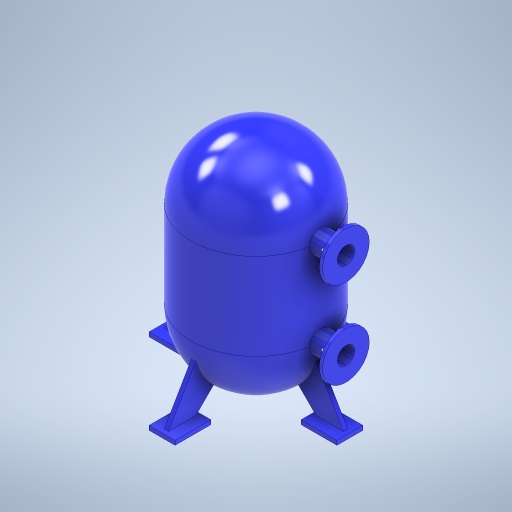
# Autodesk Inventor part: Tank
Saved by Autodesk Inventor 2023 (Build 270158000, 158)
## iProperties
Created: 2024-11-19
Part Number: Tank
Material: Generisch
Document SubType Name: Modeling
Designer: aurich
Density: 1 g/cm^3
Appearance: Vorgabe
Author: aurich
Autodesk Inventor part; units mm, degrees
ref_plane "XZ Plane" through (0, 0, 0) normal (0, 1, 0) x (-1, 0, 0)
sketch "Skizze1" plane through (0, 0, 0) normal (1, 0, 0) x (0, 1, 0)
  line L0 (0, 0) -> (1000, 0)
  line L1 (1000, 0) -> (1000, 0)
  line L2 (700, -300) -> (300, -300)
  line L3 (0, 0) -> (0, 0)
  arc A0 (700, -300) -> (1000, 0) centre (700, 0) ccw
  arc A1 (0, 0) -> (300, -300) centre (300, 0) ccw
  point P0 (1000, -300)
  dimension "d0" = 1000
  dimension "d1" = 300
  dimension "d2" = 300
  dimension "d3" = 300
  constraints: 8 end point, 4 point on circle, 4 tangent, 2 centre point, 2 perpendicular, 2 point on line, 1 horizontal, 1 vertical
  measures "d0" distance of L0.start L0.end
  measures "d1" distance of L0.end point (1000, -300)
  measures "d2" radius of A0
  measures "d3" radius of A1
revolve "Umdrehung1" add sketch "Skizze1" angle 360 about axis through (0, 0, 0) along (0, 1, 0)
sketch "Skizze2" plane through (0, 0, 0) normal (1, 0, 0) x (0, 1, 0)
  line L0 (0, 413.6092) -> (0, 288.6092)
  line L1 (0, 288.6092) -> (82.249, 206.3602)
  arc A0 (300, 300) -> (300, -300) centre (300, 0) ccw projected
  line L2 (0, 413.6092) -> (217.0398, 288.3012)
  line L3 (0, 413.6092) -> (250.616, 413.6092) construction
  line L4 (217.0398, 288.3012) -> (237.0888, 275.082)
  line L5 (237.0888, 275.082) -> (125.308, 163.3012)
  line L6 (82.249, 206.3602) -> (125.308, 163.3012)
  point P0 (0, 0)
  point P1 (0, 0)
  dimension "d5" = 125
  dimension "d6" = 135
  dimension "d7" = 30
  constraints: 14 end point, 3 point on circle, 1 equal length, 1 horizontal, 1 perpendicular, 1 point on line, 1 vertical, 1 vertical alignment
  measures "d5" distance of L0.start L0.end
  measures "d6" angle of L1 L0
  measures "d7" angle of L2 L3
extrude "Extrusion1" add sketch "Skizze2" along normal mid plane 20
sketch "Skizze3" plane through (-10, 0, 288.6092) normal (0, -1, 0) x (1, 0, 0)
  line L0 (-50, -20) -> (70, -20)
  line L1 (70, -20) -> (70, 145)
  line L2 (70, 145) -> (-50, 145)
  line L3 (-50, 145) -> (-50, -20)
  line L4 (0, 125) -> (20, 125) projected
  line L5 (20, 0) -> (0, 0) projected
  line L6 (20, 125) -> (20, 0) projected
  line L7 (0, 0) -> (0, 125) projected
  point P0 (10, -288.6092)
  dimension "d10" = 20
  dimension "d11" = 20
  dimension "d12" = 50
  dimension "d13" = 50
  constraints: 8 end point, 2 parallel, 1 horizontal, 1 perpendicular
  measures "d10" distance between parallel lines of L4 L2
  measures "d11" distance between parallel lines of L5 L0
  measures "d12" distance between parallel lines of L1 L6
  measures "d13" distance between parallel lines of L7 L3
extrude "Extrusion2" add sketch "Skizze3" along normal blind 20 contours L3 L2 L1 L0 | L4 L6 L5 L7
pattern_circular "Runde Anordnung1" count 4 over 360 about axis through (0, -10, 0) along (0, 1, 0) of "Extrusion1", "Extrusion2"
ref_plane "Arbeitsebene1" through (300, 500, 0) normal (1, 0, 0) x (0, 1, 0)
sketch "Skizze4" plane through (300, 500, 0) normal (1, 0, 0) x (0, 1, 0)
  circle A0 centre (-200, 0) radius 40
  circle A1 centre (-200, 0) radius 50
  line L0 (-200, -300) -> (-200, 300) projected
  point P0 (-500, 0)
  dimension "d20" = 100
  constraints: 3 coincident, 2 centre point, 1 midpoint
  measures "d20" diameter of A1
extrude "Extrusion3" add sketch "Skizze4" along normal mid plane 200 contours A0 L0 A1 | A0 L0 A1
sketch "Skizze5" plane through (400, 300, 0) normal (1, 0, 0) x (0, 0, -1)
  circle A0 centre (0, 0) radius 40
  circle A1 centre (0, 0) radius 108
  point P0 (0, -300)
  dimension "d23" = 216
  dimension "d24" = 80
  constraints: 2 centre point, 2 coincident
  measures "d23" diameter of A1
  measures "d24" diameter of A0
extrude "Extrusion4" add sketch "Skizze5" along normal blind 15
sketch "Skizze6" plane through (400, 300, 0) normal (-1, 0, 0) x (0, 0, 1)
  circle A0 centre (0, -85) radius 10 construction
  line L0 (0, -95) -> (-8.7647, -89.8146)
  line L1 (-8.7647, -80.1854) -> (0, -75)
  line L2 (0, -75) -> (8.7647, -80.1854)
  line L3 (8.7647, -80.1854) -> (8.7647, -89.8146)
  line L4 (0, -95) -> (8.7647, -89.8146)
  line L5 (-8.7647, -80.1854) -> (-8.7647, -89.8146)
  circle A1 centre (0, 0) radius 40 projected
  point P0 (0, -300)
  dimension "d27" = 20
  dimension "d28" = 85
  constraints: 12 end point, 6 point on circle, 2 horizontal alignment, 2 parallel, 1 centre point, 1 vertical, 1 vertical alignment
  measures "d27" diameter of A0
  measures "d28" distance of A1.centre A0.centre
extrude "Extrusion5" add sketch "Skizze6" along normal blind 10 contours L0 L5 L1 L2 L3 L4
sketch "Skizze7" plane through (390, 300, 0) normal (-1, 0, 0) x (0, 0, 1)
  circle A0 centre (0, -85) radius 5
  point P0 (0, -300)
  dimension "d31" = 10
  constraints: 1 centre point
  measures "d31" diameter of A0
extrude "Extrusion6" add sketch "Skizze7" along normal blind 10
pattern_circular "Runde Anordnung2" count 6 over 360 about axis through (300, 300, 0) along (1, 0, 0) of "Extrusion5", "Extrusion6"
ref_plane "Arbeitsebene2" through (-10, 500, 288.6092) normal (0, -1, 0) x (1, 0, 0)
mirror "Spiegeln1" about plane through (-10, 500, 288.6092) normal (0, -1, 0) of "Extrusion3", "Extrusion4"
mirror "Spiegeln2" about plane through (-10, 500, 288.6092) normal (0, -1, 0) of "Extrusion5", "Extrusion6", "Runde Anordnung2"
equation "\"d11\" = d10"
